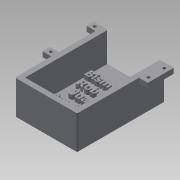
# Autodesk Inventor part: Cover Batera 2i
Saved by Autodesk Inventor 2015 SP1 (Build 190203100, 203)
## iProperties
Created: 2015-03-25
Part Number: Cover Batera 2i
Material: Generic
Document SubType Name: Modeling
Designer: Rafi Kurnia Putra
Density: 1 g/cm^3
Appearance: Default
Author: Rafi Kurnia Putra
Autodesk Inventor part; units mm, degrees
(part 1 of 2)
ref_plane "YZ Plane" through (0, 0, 0) normal (1, 0, 0) x (0, 1, 0)
ref_plane "XZ Plane" through (0, 0, 0) normal (0, 1, 0) x (-1, 0, 0)
ref_plane "XY Plane" through (0, 0, 0) normal (0, 0, 1) x (1, 0, 0)
sketch "Sketch1" plane through (0, 0, 0) normal (0, 0, 1) x (1, 0, 0)
  line L0 (-21.25, -30) -> (21.25, -30)
  line L1 (21.25, -30) -> (21.25, 30)
  line L2 (21.25, 30) -> (-21.25, 30)
  line L3 (-21.25, 30) -> (-21.25, -30)
  line L4 (-21.25, -30) -> (21.25, 30) construction
  line L5 (21.25, -30) -> (-21.25, 30) construction
  point P0 (0, 0)
  dimension "d0" = 42.5
  dimension "d1" = 60
  constraints: 12 end point, 2 midpoint, 2 parallel, 1 horizontal, 1 perpendicular
  measures "d0" distance of L2.end L1.end
  measures "d1" distance of L1.end L0.end
extrude "Extrusion1" add sketch "Sketch1" along normal blind 3.5
sketch "Sketch4" plane through (0, 0, 3.5) normal (0, 0, 1) x (1, 0, 0)
  line L0 (-21.25, -30) -> (21.25, -30) projected
  line L1 (-21.25, 30) -> (-17.75, 30)
  line L2 (-17.75, 30) -> (-17.75, -26.5)
  line L3 (-19, -30) -> (-21.25, -30)
  line L4 (-21.25, -30) -> (-21.25, 30)
  line L5 (21.25, 30) -> (17.75, 30)
  line L6 (17.75, 30) -> (17.75, -26.5)
  line L7 (19, -30) -> (21.25, -30)
  line L8 (21.25, -30) -> (21.25, 30)
  line L9 (19, -30) -> (-19, -30)
  line L10 (-17.75, -26.5) -> (17.75, -26.5)
  point P0 (0, 0)
  dimension "d23" = 3.5
  constraints: 20 end point, 5 parallel, 4 horizontal, 3 vertical, 2 perpendicular, 2 point on line
  measures "d23" distance between parallel lines of L8 L6
extrude "Extrusion3" add sketch "Sketch4" along normal blind 20
sketch "Sketch5" plane through (0, 0, 23.5) normal (0, 0, 1) x (1, 0, 0)
  line L0 (-21.25, 30) -> (-27.25, 30)
  line L1 (-27.25, 30) -> (-27.25, -30)
  line L2 (-27.25, -30) -> (-21.25, -30)
  line L3 (-21.25, -30) -> (-21.25, 30)
  line L4 (21.25, 30) -> (27.25, 30)
  line L5 (27.25, 30) -> (27.25, -30)
  line L6 (27.25, -30) -> (21.25, -30)
  line L7 (21.25, -30) -> (21.25, 30)
  point P0 (0, 0)
  dimension "d21" = 6
  dimension "d22" = 6
  constraints: 16 end point, 4 parallel, 2 horizontal, 2 perpendicular, 1 point on line
  measures "d21" distance of L4.start L4.end
  measures "d22" distance of L0.start L0.end
extrude "Extrusion4" add sketch "Sketch5" against normal blind 3.5
sketch "Sketch6" plane through (0, 0, 20) normal (0, 0, -1) x (-1, 0, 0)
  line L0 (-27.25, 30) -> (-27.25, -30) projected
  line L1 (-21.25, -30) -> (-21.25, 30) projected
  line L2 (-27.25, 25) -> (-21.25, 25)
  line L3 (-21.25, 25) -> (-21.25, 0)
  line L4 (-21.25, 0) -> (-27.25, 0)
  line L5 (-27.25, 0) -> (-27.25, 25)
  point P0 (0, 0)
  constraints: 8 end point, 2 parallel, 1 horizontal, 1 midpoint, 1 perpendicular, 1 point on line
extrude "Extrusion5" cut sketch "Sketch6" against normal up to next
sketch "Sketch7" plane through (0, 0, 20) normal (0, 0, -1) x (-1, 0, 0)
  line L0 (21.25, 12.215) -> (41.1215, 12.215) projected
  line L1 (27.25, -30) -> (27.25, 30) projected
  line L2 (27.25, 12.215) -> (21.25, 12.215)
  line L3 (21.25, 12.215) -> (21.25, -30)
  line L4 (21.25, -30) -> (27.25, -30)
  line L5 (27.25, -30) -> (27.25, 12.215)
  point P0 (0, 0)
  constraints: 8 end point, 2 parallel, 2 point on line, 1 horizontal, 1 perpendicular
extrude "Extrusion6" cut sketch "Sketch7" against normal up to next
sketch "Sketch8" plane through (0, 0, 20) normal (0, 0, -1) x (-1, 0, 0)
  line L0 (-29.9641, -5.0076) -> (-82.628, -5.0076) projected
  line L1 (-27.25, 0) -> (-27.25, -30) projected
  line L2 (-27.25, -5.0076) -> (-21.25, -5.0076)
  line L3 (-21.25, -5.0076) -> (-21.25, -30)
  line L4 (-21.25, -30) -> (-27.25, -30)
  line L5 (-27.25, -30) -> (-27.25, -5.0076)
  point P0 (0, 0)
  constraints: 8 end point, 2 parallel, 1 horizontal, 1 perpendicular, 1 point on line
extrude "Extrusion7" cut sketch "Sketch8" against normal up to next
sketch "Sketch11" plane through (0, 0, 20) normal (0, 0, -1) x (-1, 0, 0)
  line L0 (-27.25, 25) -> (-21.25, 25) projected
  line L1 (-21.25, 30) -> (-21.25, 25) projected
  line L2 (-21.25, 30) -> (-27.25, 30) projected
  line L3 (-27.25, 30) -> (-27.25, 25) projected
  line L4 (-27.25, -5.0076) -> (-21.25, -5.0076) projected
  line L5 (-21.25, 0) -> (-21.25, -5.0076) projected
  line L6 (-21.25, 0) -> (-27.25, 0) projected
  line L7 (-27.25, 0) -> (-27.25, -5.0076) projected
  line L8 (21.25, 12.215) -> (27.25, 12.215) projected
  line L9 (27.25, 12.215) -> (27.25, 30) projected
  line L10 (27.25, 30) -> (21.25, 30) projected
  line L11 (21.25, 12.215) -> (21.25, 30) projected
  circle A0 centre (-24.25, 27.5) radius 1
  circle A1 centre (-24.25, -2.5038) radius 1
  circle A2 centre (24.25, 26.5) radius 1
  circle A3 centre (24.25, 15.715) radius 1
  point P0 (0, 0)
  dimension "d24" = 2
  dimension "d25" = 2
  dimension "d26" = 2
  dimension "d27" = 2
  dimension "d28" = 3.5
  constraints: 4 centre point
  measures "d24" diameter of A0
  measures "d25" diameter of A1
  measures "d26" diameter of A2
  measures "d27" diameter of A3
  measures "d28" distance from line of L8 A3.centre
extrude "Extrusion8" cut sketch "Sketch11" against normal up to next contours A0 | A1 | A2 | A3
fillet "Fillet1" radius 1 8 edges at (-21.25, 0, 0) (21.25, 0, 0) (0, -30, 0) (-21.25, -30, 11.75) (21.25, -30, 11.75) (0, 30, 0) (-21.25, 30, 10) (21.25, 30, 10)
sketch "Sketch12" plane through (0, 0, 0) normal (0, 0, -1) x (-1, 0, 0)
  line L0 (-18.2931, -19.3693) -> (18.2839, -19.3693) construction
  line L1 (18.2839, -19.3693) -> (18.2839, -25.7267) construction
  line L2 (18.2839, -25.7267) -> (-18.2931, -25.7267) construction
  line L3 (-18.2931, -25.7267) -> (-18.2931, -19.3693) construction
  line L4 (-11.5666, -25.048) -> (-13.0942, -25.048)
  line L5 (-13.0942, -25.048) -> (-14.484, -23.2125)
  line L6 (-14.484, -23.2125) -> (-14.9378, -23.2125)
  line L7 (-14.9378, -23.2125) -> (-14.9378, -25.048)
  line L8 (-14.9378, -25.048) -> (-16.1858, -25.048)
  line L9 (-16.1858, -25.048) -> (-16.1858, -20.048)
  line L10 (-16.1858, -20.048) -> (-14.176, -20.048)
  spline S0 degree 2 poles (-14.176, -20.048) (-13.7587, -20.048) (-13.1428, -20.1533) (-12.8794, -20.3154) knots 0 0 0 1 2 2 2
  spline S1 degree 2 poles (-12.8794, -20.3154) (-12.612, -20.4856) (-12.296, -21.0164) (-12.296, -21.4216) knots 0 0 0 1 2 2 2
  spline S2 degree 2 poles (-12.296, -21.4216) (-12.296, -21.9929) (-12.8146, -22.7101) (-13.2482, -22.9208) knots 0 0 0 1 2 2 2
  line L11 (-13.2482, -22.9208) -> (-11.5666, -25.048)
  spline S3 degree 2 poles (-13.5845, -21.5796) (-13.5845, -21.3892) (-13.7303, -21.1177) (-13.8965, -21.0447) knots 0 0 0 1 2 2 2
  spline S4 degree 2 poles (-13.8965, -21.0447) (-14.014, -20.9961) (-14.3016, -20.9678) (-14.5164, -20.9678) knots 0 0 0 1 2 2 2
  line L12 (-14.5164, -20.9678) -> (-14.9378, -20.9678)
  line L13 (-14.9378, -20.9678) -> (-14.9378, -22.313)
  line L14 (-14.9378, -22.313) -> (-14.5772, -22.313)
  spline S5 degree 2 poles (-14.5772, -22.313) (-14.3178, -22.313) (-13.9491, -22.2482) (-13.8235, -22.1469) knots 0 0 0 1 2 2 2
  spline S6 degree 2 poles (-13.8235, -22.1469) (-13.702, -22.0496) (-13.5845, -21.7903) (-13.5845, -21.5796) knots 0 0 0 1 2 2 2
  spline S7 degree 2 poles (-6.6436, -22.548) (-6.6436, -23.7636) (-7.9402, -25.1533) (-9.0666, -25.1533) knots 0 0 0 1 2 2 2
  spline S8 degree 2 poles (-9.0666, -25.1533) (-10.1971, -25.1533) (-11.4856, -23.7473) (-11.4856, -22.548) knots 0 0 0 1 2 2 2
  spline S9 degree 2 poles (-11.4856, -22.548) (-11.4856, -21.3446) (-10.1971, -19.9426) (-9.0666, -19.9426) knots 0 0 0 1 2 2 2
  spline S10 degree 2 poles (-9.0666, -19.9426) (-7.9402, -19.9426) (-6.6436, -21.3365) (-6.6436, -22.548) knots 0 0 0 1 2 2 2
  spline S11 degree 2 poles (-7.9402, -22.548) (-7.9402, -22.0982) (-8.1225, -21.4702) (-8.2806, -21.2717) knots 0 0 0 1 2 2 2
  spline S12 degree 2 poles (-8.2806, -21.2717) (-8.4386, -21.065) (-8.8438, -20.8867) (-9.0626, -20.8867) knots 0 0 0 1 2 2 2
  spline S13 degree 2 poles (-9.0626, -20.8867) (-9.2935, -20.8867) (-9.6704, -21.0529) (-9.8446, -21.2636) knots 0 0 0 1 2 2 2
  spline S14 degree 2 poles (-9.8446, -21.2636) (-9.9986, -21.458) (-10.189, -22.1023) (-10.189, -22.548) knots 0 0 0 1 2 2 2
  spline S15 degree 2 poles (-10.189, -22.548) (-10.189, -23.0099) (-10.0067, -23.6177) (-9.8486, -23.8243) knots 0 0 0 1 2 2 2
  spline S16 degree 2 poles (-9.8486, -23.8243) (-9.6906, -24.031) (-9.2814, -24.2093) (-9.0626, -24.2093) knots 0 0 0 1 2 2 2
  spline S17 degree 2 poles (-9.0626, -24.2093) (-8.8397, -24.2093) (-8.4264, -24.0188) (-8.2765, -23.8162) knots 0 0 0 1 2 2 2
  spline S18 degree 2 poles (-8.2765, -23.8162) (-8.1144, -23.5974) (-7.9402, -23.018) (-7.9402, -22.548) knots 0 0 0 1 2 2 2
  spline S19 degree 2 poles (-1.9029, -23.5164) (-1.9029, -23.8892) (-2.1866, -24.4524) (-2.4216, -24.6388) knots 0 0 0 1 2 2 2
  spline S20 degree 2 poles (-2.4216, -24.6388) (-2.7052, -24.8616) (-3.3778, -25.048) (-3.9005, -25.048) knots 0 0 0 1 2 2 2
  line L15 (-3.9005, -25.048) -> (-5.8981, -25.048)
  line L16 (-5.8981, -25.048) -> (-5.8981, -20.048)
  line L17 (-5.8981, -20.048) -> (-4.1355, -20.048)
  spline S21 degree 2 poles (-4.1355, -20.048) (-3.5845, -20.048) (-3.0172, -20.1331) (-2.77, -20.2668) knots 0 0 0 1 2 2 2
  spline S22 degree 2 poles (-2.77, -20.2668) (-2.4986, -20.4086) (-2.2352, -20.8948) (-2.2352, -21.2109) knots 0 0 0 1 2 2 2
  spline S23 degree 2 poles (-2.2352, -21.2109) (-2.2352, -21.5755) (-2.5999, -22.1469) (-2.924, -22.2806) knots 0 0 0 1 2 2 2
  line L18 (-2.924, -22.2806) -> (-2.924, -22.3049)
  spline S24 degree 2 poles (-2.924, -22.3049) (-2.458, -22.4021) (-1.9029, -23.0059) (-1.9029, -23.5164) knots 0 0 0 1 2 2 2
  spline S25 degree 2 poles (-3.1995, -23.4961) (-3.1995, -23.2611) (-3.3859, -22.9977) (-3.5723, -22.9289) knots 0 0 0 1 2 2 2
  spline S26 degree 2 poles (-3.5723, -22.9289) (-3.6858, -22.8843) (-4.0869, -22.8762) (-4.4191, -22.8762) knots 0 0 0 1 2 2 2
  line L19 (-4.4191, -22.8762) -> (-4.6501, -22.8762)
  line L20 (-4.6501, -22.8762) -> (-4.6501, -24.1363)
  line L21 (-4.6501, -24.1363) -> (-4.5812, -24.1363)
  spline S27 degree 2 poles (-4.5812, -24.1363) (-4.095, -24.1363) (-3.7222, -24.1242) (-3.5277, -24.0391) knots 0 0 0 1 2 2 2
  spline S28 degree 2 poles (-3.5277, -24.0391) (-3.3576, -23.9621) (-3.1995, -23.6785) (-3.1995, -23.4961) knots 0 0 0 1 2 2 2
  spline S29 degree 2 poles (-3.5115, -21.458) (-3.5115, -21.3365) (-3.6371, -21.0812) (-3.7668, -21.0245) knots 0 0 0 1 2 2 2
  spline S30 degree 2 poles (-3.7668, -21.0245) (-3.8883, -20.9678) (-4.2287, -20.9597) (-4.565, -20.9597) knots 0 0 0 1 2 2 2
  line L22 (-4.565, -20.9597) -> (-4.6501, -20.9597)
  line L23 (-4.6501, -20.9597) -> (-4.6501, -22.0212)
  line L24 (-4.6501, -22.0212) -> (-4.4921, -22.0212)
  spline S31 degree 2 poles (-4.4921, -22.0212) (-4.172, -22.0212) (-3.9127, -22.0091) (-3.7749, -21.9443) knots 0 0 0 1 2 2 2
  spline S32 degree 2 poles (-3.7749, -21.9443) (-3.625, -21.8713) (-3.5115, -21.6242) (-3.5115, -21.458) knots 0 0 0 1 2 2 2
  spline S33 degree 2 poles (0.8402, -25.1533) (-0.1687, -25.1533) (-1.2546, -24.1809) (-1.2546, -23.2409) knots 0 0 0 1 2 2 2
  line L25 (-1.2546, -23.2409) -> (-1.2546, -20.048)
  line L26 (-1.2546, -20.048) -> (0.0014, -20.048)
  line L27 (0.0014, -20.048) -> (0.0014, -23.1679)
  spline S34 degree 2 poles (0.0014, -23.1679) (0.0014, -23.6906) (0.3945, -24.2012) (0.8402, -24.2012) knots 0 0 0 1 2 2 2
  spline S35 degree 2 poles (0.8402, -24.2012) (1.2737, -24.2012) (1.6789, -23.7109) (1.6789, -23.1679) knots 0 0 0 1 2 2 2
  line L28 (1.6789, -23.1679) -> (1.6789, -20.048)
  line L29 (1.6789, -20.048) -> (2.935, -20.048)
  line L30 (2.935, -20.048) -> (2.935, -23.2368)
  spline S36 degree 2 poles (2.935, -23.2368) (2.935, -24.1606) (1.8775, -25.1533) (0.8402, -25.1533) knots 0 0 0 1 2 2 2
  spline S37 degree 2 poles (5.4431, -25.1371) (4.8677, -25.1371) (4.0006, -24.9143) (3.6279, -24.7522) knots 0 0 0 1 2 2 2
  line L31 (3.6279, -24.7522) -> (3.6279, -23.561)
  line L32 (3.6279, -23.561) -> (3.7413, -23.561)
  spline S38 degree 2 poles (3.7413, -23.561) (4.1181, -23.8811) (5.0217, -24.2255) (5.4471, -24.2255) knots 0 0 0 1 2 2 2
  spline S39 degree 2 poles (5.4471, -24.2255) (5.5565, -24.2255) (5.9091, -24.1768) (6.0144, -24.1282) knots 0 0 0 1 2 2 2
  spline S40 degree 2 poles (6.0144, -24.1282) (6.1441, -24.0715) (6.3264, -23.8648) (6.3264, -23.6987) knots 0 0 0 1 2 2 2
  spline S41 degree 2 poles (6.3264, -23.6987) (6.3264, -23.5083) (6.0306, -23.2733) (5.828, -23.2206) knots 0 0 0 1 2 2 2
  spline S42 degree 2 poles (5.828, -23.2206) (5.5728, -23.1517) (4.9933, -23.0342) (4.7381, -22.9451) knots 0 0 0 1 2 2 2
  spline S43 degree 2 poles (4.7381, -22.9451) (4.1587, -22.7425) (3.6562, -22.0496) (3.6562, -21.531) knots 0 0 0 1 2 2 2
  spline S44 degree 2 poles (3.6562, -21.531) (3.6562, -20.83) (4.8434, -19.9589) (5.7348, -19.9589) knots 0 0 0 1 2 2 2
  spline S45 degree 2 poles (5.7348, -19.9589) (6.1805, -19.9589) (7.0638, -20.1412) (7.4123, -20.2952) knots 0 0 0 1 2 2 2
  line L33 (7.4123, -20.2952) -> (7.4123, -21.4378)
  line L34 (7.4123, -21.4378) -> (7.3029, -21.4378)
  spline S46 degree 2 poles (7.3029, -21.4378) (7.0233, -21.1987) (6.2211, -20.8705) (5.7997, -20.8705) knots 0 0 0 1 2 2 2
  spline S47 degree 2 poles (5.7997, -20.8705) (5.6335, -20.8705) (5.3742, -20.9191) (5.2283, -20.984) knots 0 0 0 1 2 2 2
  spline S48 degree 2 poles (5.2283, -20.984) (5.1108, -21.0366) (4.9407, -21.2473) (4.9407, -21.377) knots 0 0 0 1 2 2 2
  spline S49 degree 2 poles (4.9407, -21.377) (4.9407, -21.5715) (5.2121, -21.7943) (5.6011, -21.8835) knots 0 0 0 1 2 2 2
  spline S50 degree 2 poles (5.6011, -21.8835) (5.8523, -21.9402) (6.3183, -22.0496) (6.5857, -22.1428) knots 0 0 0 1 2 2 2
  spline S51 degree 2 poles (6.5857, -22.1428) (7.1044, -22.3332) (7.6108, -22.9653) (7.6108, -23.484) knots 0 0 0 1 2 2 2
  spline S52 degree 2 poles (7.6108, -23.484) (7.6108, -24.2295) (6.4399, -25.1371) (5.4431, -25.1371) knots 0 0 0 1 2 2 2
  line L35 (9.2154, -25.048) -> (9.2154, -21.0002)
  line L36 (9.2154, -21.0002) -> (7.7365, -21.0002)
  line L37 (7.7365, -21.0002) -> (7.7365, -20.048)
  line L38 (7.7365, -20.048) -> (11.9504, -20.048)
  line L39 (11.9504, -20.048) -> (11.9504, -21.0002)
  line L40 (11.9504, -21.0002) -> (10.4715, -21.0002)
  line L41 (10.4715, -21.0002) -> (10.4715, -25.048)
  line L42 (10.4715, -25.048) -> (9.2154, -25.048)
  line L43 (11.9261, -25.048) -> (13.6157, -20.048)
  line L44 (13.6157, -20.048) -> (14.9852, -20.048)
  line L45 (14.9852, -20.048) -> (16.6749, -25.048)
  line L46 (16.6749, -25.048) -> (15.3823, -25.048)
  line L47 (15.3823, -25.048) -> (15.0703, -24.0269)
  line L48 (15.0703, -24.0269) -> (13.4982, -24.0269)
  line L49 (13.4982, -24.0269) -> (13.1822, -25.048)
  line L50 (13.1822, -25.048) -> (11.9261, -25.048)
  line L51 (14.7948, -23.1193) -> (14.2843, -21.4661)
  line L52 (14.2843, -21.4661) -> (13.7697, -23.1193)
  line L53 (13.7697, -23.1193) -> (14.7948, -23.1193)
  point P0 (0, 0)
  constraints: 2 other
extrude "Extrusion9" cut sketch "Sketch12" against normal up to next
sketch "Sketch13" plane through (0, 0, 0) normal (0, 0, -1) x (-1, 0, 0)
  spline S0 degree 2 poles (-13.8965, -21.0447) (-14.014, -20.9961) (-14.3016, -20.9678) (-14.5164, -20.9678) knots 0 0 0 0.5 1 1 1 projected
  line L0 (-14.5164, -20.9678) -> (-14.9378, -20.9678) projected
  line L1 (-14.9378, -20.9678) -> (-14.9378, -22.313) projected
  line L2 (-14.9378, -22.313) -> (-14.5772, -22.313) projected
  spline S1 degree 2 poles (-14.5772, -22.313) (-14.3178, -22.313) (-13.9491, -22.2482) (-13.8235, -22.1469) knots 0 0 0 0.5 1 1 1 projected
  spline S2 degree 2 poles (-13.8235, -22.1469) (-13.702, -22.0496) (-13.5845, -21.7903) (-13.5845, -21.5796) knots 0 0 0 0.5 1 1 1 projected
  spline S3 degree 2 poles (-13.5845, -21.5796) (-13.5845, -21.3892) (-13.7303, -21.1177) (-13.8965, -21.0447) knots 0 0 0 0.5 1 1 1 projected
  spline S4 degree 2 poles (-8.2806, -21.2717) (-8.4386, -21.065) (-8.8438, -20.8867) (-9.0626, -20.8867) knots 0 0 0 0.5 1 1 1 projected
  spline S5 degree 2 poles (-9.0626, -20.8867) (-9.2935, -20.8867) (-9.6704, -21.0529) (-9.8446, -21.2636) knots 0 0 0 0.5 1 1 1 projected
  spline S6 degree 2 poles (-9.8446, -21.2636) (-9.9986, -21.458) (-10.189, -22.1023) (-10.189, -22.548) knots 0 0 0 0.5 1 1 1 projected
  spline S7 degree 2 poles (-10.189, -22.548) (-10.189, -23.0099) (-10.0067, -23.6177) (-9.8486, -23.8243) knots 0 0 0 0.5 1 1 1 projected
  spline S8 degree 2 poles (-9.8486, -23.8243) (-9.6906, -24.031) (-9.2814, -24.2093) (-9.0626, -24.2093) knots 0 0 0 0.5 1 1 1 projected
  spline S9 degree 2 poles (-9.0626, -24.2093) (-8.8397, -24.2093) (-8.4264, -24.0188) (-8.2765, -23.8162) knots 0 0 0 0.5 1 1 1 projected
  spline S10 degree 2 poles (-8.2765, -23.8162) (-8.1144, -23.5974) (-7.9402, -23.018) (-7.9402, -22.548) knots 0 0 0 0.5 1 1 1 projected
  spline S11 degree 2 poles (-7.9402, -22.548) (-7.9402, -22.0982) (-8.1225, -21.4702) (-8.2806, -21.2717) knots 0 0 0 0.5 1 1 1 projected
  spline S12 degree 2 poles (-3.7668, -21.0245) (-3.8883, -20.9678) (-4.2287, -20.9597) (-4.565, -20.9597) knots 0 0 0 0.5 1 1 1 projected
  line L3 (-4.565, -20.9597) -> (-4.6501, -20.9597) projected
  line L4 (-4.6501, -20.9597) -> (-4.6501, -22.0212) projected
  line L5 (-4.6501, -22.0212) -> (-4.4921, -22.0212) projected
  spline S13 degree 2 poles (-4.4921, -22.0212) (-4.172, -22.0212) (-3.9127, -22.0091) (-3.7749, -21.9443) knots 0 0 0 0.5 1 1 1 projected
  spline S14 degree 2 poles (-3.7749, -21.9443) (-3.625, -21.8713) (-3.5115, -21.6242) (-3.5115, -21.458) knots 0 0 0 0.5 1 1 1 projected
  spline S15 degree 2 poles (-3.5115, -21.458) (-3.5115, -21.3365) (-3.6371, -21.0812) (-3.7668, -21.0245) knots 0 0 0 0.5 1 1 1 projected
  spline S16 degree 2 poles (-3.5723, -22.9289) (-3.6858, -22.8843) (-4.0869, -22.8762) (-4.4191, -22.8762) knots 0 0 0 0.5 1 1 1 projected
  line L6 (-4.4191, -22.8762) -> (-4.6501, -22.8762) projected
  line L7 (-4.6501, -22.8762) -> (-4.6501, -24.1363) projected
  line L8 (-4.6501, -24.1363) -> (-4.5812, -24.1363) projected
  spline S17 degree 2 poles (-4.5812, -24.1363) (-4.095, -24.1363) (-3.7222, -24.1242) (-3.5277, -24.0391) knots 0 0 0 0.5 1 1 1 projected
  spline S18 degree 2 poles (-3.5277, -24.0391) (-3.3576, -23.9621) (-3.1995, -23.6785) (-3.1995, -23.4961) knots 0 0 0 0.5 1 1 1 projected
  spline S19 degree 2 poles (-3.1995, -23.4961) (-3.1995, -23.2611) (-3.3859, -22.9977) (-3.5723, -22.9289) knots 0 0 0 0.5 1 1 1 projected
  line L9 (14.2843, -21.4661) -> (13.7697, -23.1193) projected
  line L10 (13.7697, -23.1193) -> (14.7948, -23.1193) projected
  line L11 (14.7948, -23.1193) -> (14.2843, -21.4661) projected
  point P0 (0, 0)
  constraints: 20 other
extrude "Extrusion10" cut sketch "Sketch13" against normal up to next
fillet "Fillet2" radius 1 3 edges at (-17.75, 30, 13.5) (0, 30, 3.5) (17.75, 30, 13.5)
sketch "Sketch15" plane through (0, 0, 23.5) normal (0, 0, 1) x (1, 0, 0)
  circle A0 centre (-24.25, 15.715) radius 1 projected
  circle A1 centre (24.25, -2.5038) radius 1 projected
  circle A2 centre (24.25, 27.5) radius 1 projected
  circle A3 centre (-24.25, 26.5) radius 1 projected
  arc A4 (18.75, 30) -> (17.75, 29) centre (18.75, 29) ccw projected
  line L0 (17.75, 29) -> (17.75, -26.5) projected
  line L1 (17.75, -26.5) -> (-17.75, -26.5) projected
  line L2 (-17.75, -26.5) -> (-17.75, 29) projected
  arc A5 (-17.75, 29) -> (-18.75, 30) centre (-18.75, 29) ccw projected
  line L3 (-18.75, 30) -> (-27.25, 30) projected
  line L4 (-27.25, 30) -> (-27.25, 12.215) projected
  line L5 (-27.25, 12.215) -> (-21.25, 12.215) projected
  line L6 (-21.25, 12.215) -> (-21.25, -29) projected
  arc A6 (-21.25, -29) -> (-20.25, -30) centre (-20.25, -29) ccw projected
  line L7 (-20.25, -30) -> (20.25, -30) projected
  arc A7 (20.25, -30) -> (21.25, -29) centre (20.25, -29) ccw projected
  line L8 (21.25, -29) -> (21.25, -5.0076) projected
  line L9 (21.25, -5.0076) -> (27.25, -5.0076) projected
  line L10 (27.25, 0) -> (27.25, -5.0076) projected
  line L11 (27.25, 0) -> (21.25, 0) projected
  line L12 (21.25, 0) -> (21.25, 25) projected
  line L13 (21.25, 25) -> (27.25, 25) projected
  line L14 (27.25, 30) -> (27.25, 25) projected
  line L15 (18.75, 30) -> (27.25, 30) projected
  point P0 (0, 0)
extrude "Extrusion11" cut sketch "Sketch15" against normal blind 3.5
sketch "Sketch16" plane through (0, 0, 20) normal (0, 0, 1) x (1, 0, 0)
  line L0 (-27.25, 0) -> (-21.25, 0)
  line L1 (-21.25, -5.0076) -> (-27.25, -5.0076)
  line L2 (-27.25, 0) -> (-27.25, -5.0076)
  circle A0 centre (-24.25, -2.5038) radius 1
  line L3 (-21.25, 0) -> (-21.25, 25)
  line L4 (-17.75, 29) -> (-17.75, -26.5)
  line L5 (17.75, -26.5) -> (17.75, 29)
  line L6 (-21.25, -29) -> (-21.25, -5.0076)
  arc A1 (-21.25, -29) -> (-20.25, -30) centre (-20.25, -29) ccw
  line L7 (21.25, 12.215) -> (21.25, -29)
  line L8 (-17.75, -26.5) -> (17.75, -26.5)
  line L9 (20.25, -30) -> (-20.25, -30)
  arc A2 (-17.75, 29) -> (-18.75, 30) centre (-18.75, 29) ccw
  line L10 (-21.25, 25) -> (-27.25, 25)
  circle A3 centre (-24.25, 27.5) radius 1
  line L11 (-18.75, 30) -> (-27.25, 30)
  line L12 (-27.25, 30) -> (-27.25, 25)
  arc A4 (20.25, -30) -> (21.25, -29) centre (20.25, -29) ccw
  circle A5 centre (24.25, 26.5) radius 1
  circle A6 centre (24.25, 15.715) radius 1
  line L13 (27.25, 12.215) -> (21.25, 12.215)
  line L14 (27.25, 30) -> (27.25, 12.215)
  line L15 (18.75, 30) -> (27.25, 30)
  arc A7 (18.75, 30) -> (17.75, 29) centre (18.75, 29) ccw
  point P0 (0, 0)
  constraints: 32 end point, 8 centre point, 8 point on circle
extrude "Extrusion12" add sketch "Sketch16" along normal blind 3.5
sketch "Sketch17" plane through (17.75, -26.5, 3.5) normal (-1, 0, 0) x (0, 0, 1)
  point P0 (-3.5, 26.5)
sketch "Sketch19" plane through (0, 0, 3.5) normal (0, 0, 1) x (1, 0, 0)
  line L0 (-10.8355, 3.968) -> (10.329, 3.968) construction
  line L1 (10.329, 3.968) -> (10.329, 0.2383) construction
  line L2 (10.329, 0.2383) -> (-10.8355, 0.2383) construction
  line L3 (-10.8355, 0.2383) -> (-10.8355, 3.968) construction
  spline S0 degree 2 poles (-12.6256, 14.0607) (-12.6256, 13.6879) (-12.9093, 13.1247) (-13.1443, 12.9383) knots 0 0 0 1 2 2 2
  spline S1 degree 2 poles (-13.1443, 12.9383) (-13.4279, 12.7155) (-14.1005, 12.5291) (-14.6232, 12.5291) knots 0 0 0 1 2 2 2
  line L4 (-14.6232, 12.5291) -> (-16.6208, 12.5291)
  line L5 (-16.6208, 12.5291) -> (-16.6208, 17.5291)
  line L6 (-16.6208, 17.5291) -> (-14.8582, 17.5291)
  spline S2 degree 2 poles (-14.8582, 17.5291) (-14.3071, 17.5291) (-13.7399, 17.444) (-13.4927, 17.3103) knots 0 0 0 1 2 2 2
  spline S3 degree 2 poles (-13.4927, 17.3103) (-13.2212, 17.1685) (-12.9579, 16.6822) (-12.9579, 16.3662) knots 0 0 0 1 2 2 2
  spline S4 degree 2 poles (-12.9579, 16.3662) (-12.9579, 16.0015) (-13.3225, 15.4302) (-13.6467, 15.2965) knots 0 0 0 1 2 2 2
  line L7 (-13.6467, 15.2965) -> (-13.6467, 15.2722)
  spline S5 degree 2 poles (-13.6467, 15.2722) (-13.1807, 15.1749) (-12.6256, 14.5712) (-12.6256, 14.0607) knots 0 0 0 1 2 2 2
  spline S6 degree 2 poles (-13.9222, 14.0809) (-13.9222, 14.316) (-14.1086, 14.5793) (-14.295, 14.6482) knots 0 0 0 1 2 2 2
  spline S7 degree 2 poles (-14.295, 14.6482) (-14.4084, 14.6928) (-14.8096, 14.7009) (-15.1418, 14.7009) knots 0 0 0 1 2 2 2
  line L8 (-15.1418, 14.7009) -> (-15.3728, 14.7009)
  line L9 (-15.3728, 14.7009) -> (-15.3728, 13.4407)
  line L10 (-15.3728, 13.4407) -> (-15.3039, 13.4407)
  spline S8 degree 2 poles (-15.3039, 13.4407) (-14.8177, 13.4407) (-14.4449, 13.4529) (-14.2504, 13.538) knots 0 0 0 1 2 2 2
  spline S9 degree 2 poles (-14.2504, 13.538) (-14.0802, 13.615) (-13.9222, 13.8986) (-13.9222, 14.0809) knots 0 0 0 1 2 2 2
  spline S10 degree 2 poles (-14.2342, 16.119) (-14.2342, 16.2406) (-14.3598, 16.4959) (-14.4895, 16.5526) knots 0 0 0 1 2 2 2
  spline S11 degree 2 poles (-14.4895, 16.5526) (-14.611, 16.6093) (-14.9514, 16.6174) (-15.2877, 16.6174) knots 0 0 0 1 2 2 2
  line L11 (-15.2877, 16.6174) -> (-15.3728, 16.6174)
  line L12 (-15.3728, 16.6174) -> (-15.3728, 15.5558)
  line L13 (-15.3728, 15.5558) -> (-15.2148, 15.5558)
  spline S12 degree 2 poles (-15.2148, 15.5558) (-14.8947, 15.5558) (-14.6353, 15.568) (-14.4976, 15.6328) knots 0 0 0 1 2 2 2
  spline S13 degree 2 poles (-14.4976, 15.6328) (-14.3477, 15.7057) (-14.2342, 15.9529) (-14.2342, 16.119) knots 0 0 0 1 2 2 2
  line L14 (-10.7982, 12.5291) -> (-11.9733, 12.5291)
  line L15 (-11.9733, 12.5291) -> (-11.9733, 16.3014)
  line L16 (-11.9733, 16.3014) -> (-10.7982, 16.3014)
  line L17 (-10.7982, 16.3014) -> (-10.7982, 12.5291)
  line L18 (-10.7618, 16.8403) -> (-12.0057, 16.8403)
  line L19 (-12.0057, 16.8403) -> (-12.0057, 17.756)
  line L20 (-12.0057, 17.756) -> (-10.7618, 17.756)
  line L21 (-10.7618, 17.756) -> (-10.7618, 16.8403)
  spline S14 degree 2 poles (-8.752, 12.4278) (-9.1653, 12.4278) (-9.9068, 12.6101) (-10.1499, 12.7317) knots 0 0 0 1 2 2 2
  line L22 (-10.1499, 12.7317) -> (-10.1499, 13.7244)
  line L23 (-10.1499, 13.7244) -> (-10.0527, 13.7244)
  spline S15 degree 2 poles (-10.0527, 13.7244) (-9.9676, 13.6595) (-9.7529, 13.5056) (-9.5624, 13.4205) knots 0 0 0 1 2 2 2
  spline S16 degree 2 poles (-9.5624, 13.4205) (-9.3963, 13.3435) (-8.9871, 13.2341) (-8.7439, 13.2341) knots 0 0 0 1 2 2 2
  spline S17 degree 2 poles (-8.7439, 13.2341) (-8.4968, 13.2341) (-8.1159, 13.3881) (-8.1159, 13.5542) knots 0 0 0 1 2 2 2
  spline S18 degree 2 poles (-8.1159, 13.5542) (-8.1159, 13.6839) (-8.2901, 13.8216) (-8.5413, 13.8784) knots 0 0 0 1 2 2 2
  spline S19 degree 2 poles (-8.5413, 13.8784) (-8.6751, 13.9148) (-9.0843, 13.9918) (-9.2423, 14.0404) knots 0 0 0 1 2 2 2
  spline S20 degree 2 poles (-9.2423, 14.0404) (-9.688, 14.1782) (-10.1337, 14.7171) (-10.1337, 15.1587) knots 0 0 0 1 2 2 2
  spline S21 degree 2 poles (-10.1337, 15.1587) (-10.1337, 15.41) (-9.9028, 15.8557) (-9.6759, 16.0299) knots 0 0 0 1 2 2 2
  spline S22 degree 2 poles (-9.6759, 16.0299) (-9.453, 16.2001) (-8.7926, 16.4027) (-8.3752, 16.4027) knots 0 0 0 1 2 2 2
  spline S23 degree 2 poles (-8.3752, 16.4027) (-7.9781, 16.4027) (-7.3136, 16.2446) (-7.0867, 16.1352) knots 0 0 0 1 2 2 2
  line L24 (-7.0867, 16.1352) -> (-7.0867, 15.179)
  line L25 (-7.0867, 15.179) -> (-7.1799, 15.179)
  spline S24 degree 2 poles (-7.1799, 15.179) (-7.2407, 15.2276) (-7.5041, 15.3856) (-7.6256, 15.4424) knots 0 0 0 1 2 2 2
  spline S25 degree 2 poles (-7.6256, 15.4424) (-7.7755, 15.5072) (-8.1402, 15.5963) (-8.3306, 15.5963) knots 0 0 0 1 2 2 2
  spline S26 degree 2 poles (-8.3306, 15.5963) (-8.5859, 15.5963) (-8.9384, 15.4221) (-8.9384, 15.2803) knots 0 0 0 1 2 2 2
  spline S27 degree 2 poles (-8.9384, 15.2803) (-8.9384, 15.1506) (-8.7642, 15.0048) (-8.4725, 14.9318) knots 0 0 0 1 2 2 2
  spline S28 degree 2 poles (-8.4725, 14.9318) (-8.3225, 14.8954) (-7.9295, 14.8265) (-7.7472, 14.7657) knots 0 0 0 1 2 2 2
  spline S29 degree 2 poles (-7.7472, 14.7657) (-7.342, 14.636) (-6.9206, 14.1296) (-6.9206, 13.7082) knots 0 0 0 1 2 2 2
  spline S30 degree 2 poles (-6.9206, 13.7082) (-6.9206, 13.4448) (-7.1678, 12.9626) (-7.3987, 12.8006) knots 0 0 0 1 2 2 2
  spline S31 degree 2 poles (-7.3987, 12.8006) (-7.6378, 12.6223) (-8.2942, 12.4278) (-8.752, 12.4278) knots 0 0 0 1 2 2 2
  line L26 (-1.8598, 12.5291) -> (-1.8598, 14.4132)
  spline S32 degree 2 poles (-1.8598, 14.4132) (-1.8598, 14.6928) (-1.8801, 15.0737) (-1.9287, 15.1952) knots 0 0 0 1 2 2 2
  spline S33 degree 2 poles (-1.9287, 15.1952) (-1.9814, 15.3168) (-2.1921, 15.4262) (-2.3825, 15.4262) knots 0 0 0 1 2 2 2
  spline S34 degree 2 poles (-2.3825, 15.4262) (-2.5162, 15.4262) (-2.7755, 15.3087) (-2.9295, 15.1993) knots 0 0 0 1 2 2 2
  line L27 (-2.9295, 15.1993) -> (-2.9295, 12.5291)
  line L28 (-2.9295, 12.5291) -> (-4.1127, 12.5291)
  line L29 (-4.1127, 12.5291) -> (-4.1127, 14.4132)
  spline S35 degree 2 poles (-4.1127, 14.4132) (-4.1127, 14.6887) (-4.137, 15.0737) (-4.1856, 15.1952) knots 0 0 0 1 2 2 2
  spline S36 degree 2 poles (-4.1856, 15.1952) (-4.2383, 15.3168) (-4.449, 15.4262) (-4.6394, 15.4262) knots 0 0 0 1 2 2 2
  spline S37 degree 2 poles (-4.6394, 15.4262) (-4.7812, 15.4262) (-5.0608, 15.2925) (-5.1905, 15.1993) knots 0 0 0 1 2 2 2
  line L30 (-5.1905, 15.1993) -> (-5.1905, 12.5291)
  line L31 (-5.1905, 12.5291) -> (-6.3655, 12.5291)
  line L32 (-6.3655, 12.5291) -> (-6.3655, 16.3014)
  line L33 (-6.3655, 16.3014) -> (-5.1905, 16.3014)
  line L34 (-5.1905, 16.3014) -> (-5.1905, 15.884)
  spline S38 degree 2 poles (-5.1905, 15.884) (-4.9028, 16.1271) (-4.3882, 16.4027) (-4.0681, 16.4027) knots 0 0 0 1 2 2 2
  spline S39 degree 2 poles (-4.0681, 16.4027) (-3.7237, 16.4027) (-3.1969, 16.0745) (-3.0592, 15.7463) knots 0 0 0 1 2 2 2
  spline S40 degree 2 poles (-3.0592, 15.7463) (-2.7229, 16.0623) (-2.1232, 16.4027) (-1.8153, 16.4027) knots 0 0 0 1 2 2 2
  spline S41 degree 2 poles (-1.8153, 16.4027) (-1.5519, 16.4027) (-1.1345, 16.2365) (-0.9927, 16.0664) knots 0 0 0 1 2 2 2
  spline S42 degree 2 poles (-0.9927, 16.0664) (-0.8347, 15.884) (-0.6767, 15.3856) (-0.6767, 14.9845) knots 0 0 0 1 2 2 2
  line L35 (-0.6767, 14.9845) -> (-0.6767, 12.5291)
  line L36 (-0.6767, 12.5291) -> (-1.8598, 12.5291)
  line L37 (1.3695, 12.5291) -> (0.1945, 12.5291)
  line L38 (0.1945, 12.5291) -> (0.1945, 16.3014)
  line L39 (0.1945, 16.3014) -> (1.3695, 16.3014)
  line L40 (1.3695, 16.3014) -> (1.3695, 12.5291)
  line L41 (1.406, 16.8403) -> (0.1621, 16.8403)
  line L42 (0.1621, 16.8403) -> (0.1621, 17.756)
  line L43 (0.1621, 17.756) -> (1.406, 17.756)
  line L44 (1.406, 17.756) -> (1.406, 16.8403)
  line L45 (3.4441, 12.5291) -> (2.269, 12.5291)
  line L46 (2.269, 12.5291) -> (2.269, 17.7519)
  line L47 (2.269, 17.7519) -> (3.4441, 17.7519)
  line L48 (3.4441, 17.7519) -> (3.4441, 12.5291)
  line L49 (5.5186, 12.5291) -> (4.3436, 12.5291)
  line L50 (4.3436, 12.5291) -> (4.3436, 17.7519)
  line L51 (4.3436, 17.7519) -> (5.5186, 17.7519)
  line L52 (5.5186, 17.7519) -> (5.5186, 12.5291)
  spline S43 degree 2 poles (8.4967, 12.9302) (8.3752, 12.8289) (8.1847, 12.6668) (8.0227, 12.5858) knots 0 0 0 1 2 2 2
  spline S44 degree 2 poles (8.0227, 12.5858) (7.8647, 12.5088) (7.5648, 12.4278) (7.2974, 12.4278) knots 0 0 0 1 2 2 2
  spline S45 degree 2 poles (7.2974, 12.4278) (6.795, 12.4278) (6.1345, 13.1004) (6.1345, 13.6109) knots 0 0 0 1 2 2 2
  spline S46 degree 2 poles (6.1345, 13.6109) (6.1345, 14.0283) (6.4708, 14.5469) (6.7869, 14.6968) knots 0 0 0 1 2 2 2
  spline S47 degree 2 poles (6.7869, 14.6968) (7.107, 14.8508) (7.9943, 14.9724) (8.5048, 15.0048) knots 0 0 0 1 2 2 2
  line L53 (8.5048, 15.0048) -> (8.5048, 15.025)
  spline S48 degree 2 poles (8.5048, 15.025) (8.5048, 15.337) (8.0429, 15.5761) (7.581, 15.5761) knots 0 0 0 1 2 2 2
  spline S49 degree 2 poles (7.581, 15.5761) (7.3744, 15.5761) (6.8152, 15.4262) (6.5518, 15.3087) knots 0 0 0 1 2 2 2
  line L54 (6.5518, 15.3087) -> (6.4506, 15.3087)
  line L55 (6.4506, 15.3087) -> (6.4506, 16.2203)
  spline S50 degree 2 poles (6.4506, 16.2203) (6.6248, 16.269) (7.4027, 16.4067) (7.7998, 16.4067) knots 0 0 0 1 2 2 2
  spline S51 degree 2 poles (7.7998, 16.4067) (8.7723, 16.4067) (9.6637, 15.7584) (9.6637, 15.0939) knots 0 0 0 1 2 2 2
  line L56 (9.6637, 15.0939) -> (9.6637, 12.5291)
  line L57 (9.6637, 12.5291) -> (8.4967, 12.5291)
  line L58 (8.4967, 12.5291) -> (8.4967, 12.9302)
  line L59 (8.4967, 13.5137) -> (8.4967, 14.2957)
  spline S52 degree 2 poles (8.4967, 14.2957) (8.1969, 14.2673) (7.8282, 14.2228) (7.6499, 14.1579) knots 0 0 0 1 2 2 2
  spline S53 degree 2 poles (7.6499, 14.1579) (7.4919, 14.1053) (7.3217, 13.8865) (7.3217, 13.7082) knots 0 0 0 1 2 2 2
  spline S54 degree 2 poles (7.3217, 13.7082) (7.3217, 13.4448) (7.6094, 13.2463) (7.889, 13.2463) knots 0 0 0 1 2 2 2
  spline S55 degree 2 poles (7.889, 13.2463) (8.0429, 13.2463) (8.3671, 13.3881) (8.4967, 13.5137) knots 0 0 0 1 2 2 2
  line L60 (14.064, 12.5291) -> (12.8809, 12.5291)
  line L61 (12.8809, 12.5291) -> (12.8809, 14.397)
  spline S56 degree 2 poles (12.8809, 14.397) (12.8809, 14.6279) (12.8444, 15.0818) (12.7958, 15.1871) knots 0 0 0 1 2 2 2
  spline S57 degree 2 poles (12.7958, 15.1871) (12.735, 15.3168) (12.5081, 15.4262) (12.3136, 15.4262) knots 0 0 0 1 2 2 2
  spline S58 degree 2 poles (12.3136, 15.4262) (12.1718, 15.4262) (11.876, 15.3168) (11.7099, 15.1993) knots 0 0 0 1 2 2 2
  line L62 (11.7099, 15.1993) -> (11.7099, 12.5291)
  line L63 (11.7099, 12.5291) -> (10.5348, 12.5291)
  line L64 (10.5348, 12.5291) -> (10.5348, 17.7519)
  line L65 (10.5348, 17.7519) -> (11.7099, 17.7519)
  line L66 (11.7099, 17.7519) -> (11.7099, 15.884)
  spline S59 degree 2 poles (11.7099, 15.884) (11.9976, 16.1271) (12.5446, 16.4027) (12.8768, 16.4027) knots 0 0 0 1 2 2 2
  spline S60 degree 2 poles (12.8768, 16.4027) (13.4522, 16.4027) (14.064, 15.6733) (14.064, 14.9845) knots 0 0 0 1 2 2 2
  line L67 (14.064, 14.9845) -> (14.064, 12.5291)
  line L68 (16.3614, 13.85) -> (15.1864, 11.2892)
  line L69 (15.1864, 11.2892) -> (14.4692, 11.2892)
  line L70 (14.4692, 11.2892) -> (15.1296, 13.85)
  line L71 (15.1296, 13.85) -> (16.3614, 13.85)
  line L72 (-9.3598, 4.2967) -> (-10.8874, 4.2967)
  line L73 (-10.8874, 4.2967) -> (-12.2772, 6.1322)
  line L74 (-12.2772, 6.1322) -> (-12.731, 6.1322)
  line L75 (-12.731, 6.1322) -> (-12.731, 4.2967)
  line L76 (-12.731, 4.2967) -> (-13.9789, 4.2967)
  line L77 (-13.9789, 4.2967) -> (-13.9789, 9.2967)
  line L78 (-13.9789, 9.2967) -> (-11.9692, 9.2967)
  spline S61 degree 2 poles (-11.9692, 9.2967) (-11.5519, 9.2967) (-10.936, 9.1914) (-10.6726, 9.0293) knots 0 0 0 1 2 2 2
  spline S62 degree 2 poles (-10.6726, 9.0293) (-10.4052, 8.8591) (-10.0892, 8.3283) (-10.0892, 7.9231) knots 0 0 0 1 2 2 2
  spline S63 degree 2 poles (-10.0892, 7.9231) (-10.0892, 7.3518) (-10.6078, 6.6346) (-11.0413, 6.4239) knots 0 0 0 1 2 2 2
  line L79 (-11.0413, 6.4239) -> (-9.3598, 4.2967)
  spline S64 degree 2 poles (-11.3777, 7.7651) (-11.3777, 7.9555) (-11.5235, 8.227) (-11.6896, 8.3) knots 0 0 0 1 2 2 2
  spline S65 degree 2 poles (-11.6896, 8.3) (-11.8071, 8.3486) (-12.0948, 8.3769) (-12.3096, 8.3769) knots 0 0 0 1 2 2 2
  line L80 (-12.3096, 8.3769) -> (-12.731, 8.3769)
  line L81 (-12.731, 8.3769) -> (-12.731, 7.0317)
  line L82 (-12.731, 7.0317) -> (-12.3704, 7.0317)
  spline S66 degree 2 poles (-12.3704, 7.0317) (-12.111, 7.0317) (-11.7423, 7.0965) (-11.6167, 7.1978) knots 0 0 0 1 2 2 2
  spline S67 degree 2 poles (-11.6167, 7.1978) (-11.4952, 7.2951) (-11.3777, 7.5544) (-11.3777, 7.7651) knots 0 0 0 1 2 2 2
  spline S68 degree 2 poles (-5.4376, 6.1808) (-5.4376, 5.2489) (-6.4546, 4.1792) (-7.3825, 4.1792) knots 0 0 0 1 2 2 2
  spline S69 degree 2 poles (-7.3825, 4.1792) (-8.3063, 4.1792) (-9.3315, 5.2489) (-9.3315, 6.1808) knots 0 0 0 1 2 2 2
  spline S70 degree 2 poles (-9.3315, 6.1808) (-9.3315, 7.1209) (-8.3063, 8.1865) (-7.3825, 8.1865) knots 0 0 0 1 2 2 2
  spline S71 degree 2 poles (-7.3825, 8.1865) (-6.4587, 8.1865) (-5.4376, 7.1168) (-5.4376, 6.1808) knots 0 0 0 1 2 2 2
  spline S72 degree 2 poles (-6.641, 6.1727) (-6.641, 6.509) (-6.7504, 6.9588) (-6.8477, 7.0925) knots 0 0 0 1 2 2 2
  spline S73 degree 2 poles (-6.8477, 7.0925) (-6.953, 7.2343) (-7.2164, 7.3437) (-7.3825, 7.3437) knots 0 0 0 1 2 2 2
  spline S74 degree 2 poles (-7.3825, 7.3437) (-7.5446, 7.3437) (-7.7999, 7.2465) (-7.9052, 7.1087) knots 0 0 0 1 2 2 2
  spline S75 degree 2 poles (-7.9052, 7.1087) (-8.0065, 6.979) (-8.1281, 6.5212) (-8.1281, 6.1727) knots 0 0 0 1 2 2 2
  spline S76 degree 2 poles (-8.1281, 6.1727) (-8.1281, 5.8283) (-8.0146, 5.4029) (-7.9214, 5.2732) knots 0 0 0 1 2 2 2
  spline S77 degree 2 poles (-7.9214, 5.2732) (-7.8282, 5.1436) (-7.5446, 5.022) (-7.3744, 5.022) knots 0 0 0 1 2 2 2
  spline S78 degree 2 poles (-7.3744, 5.022) (-7.2326, 5.022) (-6.9409, 5.1436) (-6.8517, 5.2651) knots 0 0 0 1 2 2 2
  spline S79 degree 2 poles (-6.8517, 5.2651) (-6.7504, 5.4069) (-6.641, 5.8162) (-6.641, 6.1727) knots 0 0 0 1 2 2 2
  spline S80 degree 2 poles (-1.1183, 6.2335) (-1.1183, 5.334) (-2.03, 4.2238) (-2.7067, 4.2238) knots 0 0 0 1 2 2 2
  spline S81 degree 2 poles (-2.7067, 4.2238) (-2.9862, 4.2238) (-3.4036, 4.3494) (-3.6386, 4.4831) knots 0 0 0 1 2 2 2
  line L83 (-3.6386, 4.4831) -> (-3.6872, 4.2967)
  line L84 (-3.6872, 4.2967) -> (-4.8136, 4.2967)
  line L85 (-4.8136, 4.2967) -> (-4.8136, 9.5196)
  line L86 (-4.8136, 9.5196) -> (-3.6386, 9.5196)
  line L87 (-3.6386, 9.5196) -> (-3.6386, 7.6719)
  spline S82 degree 2 poles (-3.6386, 7.6719) (-3.3793, 7.8948) (-2.8444, 8.1703) (-2.4919, 8.1703) knots 0 0 0 1 2 2 2
  spline S83 degree 2 poles (-2.4919, 8.1703) (-1.8315, 8.1703) (-1.1183, 7.1452) (-1.1183, 6.2335) knots 0 0 0 1 2 2 2
  spline S84 degree 2 poles (-2.3217, 6.2092) (-2.3217, 6.7724) (-2.6621, 7.2546) (-3.0187, 7.2546) knots 0 0 0 1 2 2 2
  spline S85 degree 2 poles (-3.0187, 7.2546) (-3.1767, 7.2546) (-3.4887, 7.1533) (-3.6386, 7.052) knots 0 0 0 1 2 2 2
  line L88 (-3.6386, 7.052) -> (-3.6386, 5.1638)
  spline S86 degree 2 poles (-3.6386, 5.1638) (-3.5211, 5.1152) (-3.282, 5.0828) (-3.1645, 5.0828) knots 0 0 0 1 2 2 2
  spline S87 degree 2 poles (-3.1645, 5.0828) (-2.7391, 5.0828) (-2.3217, 5.646) (-2.3217, 6.2092) knots 0 0 0 1 2 2 2
  line L89 (3.0308, 4.2967) -> (1.8557, 4.2967)
  line L90 (1.8557, 4.2967) -> (1.8557, 4.7141)
  spline S88 degree 2 poles (1.8557, 4.7141) (1.5518, 4.4588) (1.0413, 4.1914) (0.6888, 4.1914) knots 0 0 0 1 2 2 2
  spline S89 degree 2 poles (0.6888, 4.1914) (0.1296, 4.1914) (-0.4984, 4.9004) (-0.4984, 5.6136) knots 0 0 0 1 2 2 2
  line L91 (-0.4984, 5.6136) -> (-0.4984, 8.069)
  line L92 (-0.4984, 8.069) -> (0.6847, 8.069)
  line L93 (0.6847, 8.069) -> (0.6847, 6.197)
  spline S90 degree 2 poles (0.6847, 6.197) (0.6847, 5.9053) (0.7131, 5.5325) (0.7698, 5.4069) knots 0 0 0 1 2 2 2
  spline S91 degree 2 poles (0.7698, 5.4069) (0.8266, 5.2894) (1.0494, 5.1679) (1.252, 5.1679) knots 0 0 0 1 2 2 2
  spline S92 degree 2 poles (1.252, 5.1679) (1.3736, 5.1679) (1.7139, 5.2894) (1.8557, 5.3948) knots 0 0 0 1 2 2 2
  line L94 (1.8557, 5.3948) -> (1.8557, 8.069)
  line L95 (1.8557, 8.069) -> (3.0308, 8.069)
  line L96 (3.0308, 8.069) -> (3.0308, 4.2967)
  spline S93 degree 2 poles (5.077, 4.1954) (4.6637, 4.1954) (3.9222, 4.3777) (3.6791, 4.4993) knots 0 0 0 1 2 2 2
  line L97 (3.6791, 4.4993) -> (3.6791, 5.492)
  line L98 (3.6791, 5.492) -> (3.7763, 5.492)
  spline S94 degree 2 poles (3.7763, 5.492) (3.8614, 5.4272) (4.0762, 5.2732) (4.2666, 5.1881) knots 0 0 0 1 2 2 2
  spline S95 degree 2 poles (4.2666, 5.1881) (4.4327, 5.1111) (4.842, 5.0017) (5.0851, 5.0017) knots 0 0 0 1 2 2 2
  spline S96 degree 2 poles (5.0851, 5.0017) (5.3322, 5.0017) (5.7131, 5.1557) (5.7131, 5.3218) knots 0 0 0 1 2 2 2
  spline S97 degree 2 poles (5.7131, 5.3218) (5.7131, 5.4515) (5.5389, 5.5893) (5.2877, 5.646) knots 0 0 0 1 2 2 2
  spline S98 degree 2 poles (5.2877, 5.646) (5.154, 5.6824) (4.7447, 5.7594) (4.5867, 5.8081) knots 0 0 0 1 2 2 2
  spline S99 degree 2 poles (4.5867, 5.8081) (4.141, 5.9458) (3.6953, 6.4847) (3.6953, 6.9264) knots 0 0 0 1 2 2 2
  spline S100 degree 2 poles (3.6953, 6.9264) (3.6953, 7.1776) (3.9262, 7.6233) (4.1531, 7.7975) knots 0 0 0 1 2 2 2
  spline S101 degree 2 poles (4.1531, 7.7975) (4.376, 7.9677) (5.0364, 8.1703) (5.4538, 8.1703) knots 0 0 0 1 2 2 2
  spline S102 degree 2 poles (5.4538, 8.1703) (5.8509, 8.1703) (6.5154, 8.0123) (6.7423, 7.9029) knots 0 0 0 1 2 2 2
  line L99 (6.7423, 7.9029) -> (6.7423, 6.9466)
  line L100 (6.7423, 6.9466) -> (6.6491, 6.9466)
  spline S103 degree 2 poles (6.6491, 6.9466) (6.5883, 6.9953) (6.3249, 7.1533) (6.2034, 7.21) knots 0 0 0 1 2 2 2
  spline S104 degree 2 poles (6.2034, 7.21) (6.0535, 7.2748) (5.6888, 7.364) (5.4984, 7.364) knots 0 0 0 1 2 2 2
  spline S105 degree 2 poles (5.4984, 7.364) (5.2431, 7.364) (4.8906, 7.1897) (4.8906, 7.0479) knots 0 0 0 1 2 2 2
  spline S106 degree 2 poles (4.8906, 7.0479) (4.8906, 6.9183) (5.0648, 6.7724) (5.3565, 6.6995) knots 0 0 0 1 2 2 2
  spline S107 degree 2 poles (5.3565, 6.6995) (5.5065, 6.663) (5.8995, 6.5941) (6.0818, 6.5333) knots 0 0 0 1 2 2 2
  spline S108 degree 2 poles (6.0818, 6.5333) (6.487, 6.4037) (6.9084, 5.8972) (6.9084, 5.4758) knots 0 0 0 1 2 2 2
  spline S109 degree 2 poles (6.9084, 5.4758) (6.9084, 5.2124) (6.6612, 4.7303) (6.4303, 4.5682) knots 0 0 0 1 2 2 2
  spline S110 degree 2 poles (6.4303, 4.5682) (6.1912, 4.3899) (5.5348, 4.1954) (5.077, 4.1954) knots 0 0 0 1 2 2 2
  spline S111 degree 2 poles (8.91, 4.2238) (8.1929, 4.2238) (7.5364, 4.8154) (7.5364, 5.488) knots 0 0 0 1 2 2 2
  line L101 (7.5364, 5.488) -> (7.5364, 7.2505)
  line L102 (7.5364, 7.2505) -> (7.0867, 7.2505)
  line L103 (7.0867, 7.2505) -> (7.0867, 8.069)
  line L104 (7.0867, 8.069) -> (7.5364, 8.069)
  line L105 (7.5364, 8.069) -> (7.5364, 9.1468)
  line L106 (7.5364, 9.1468) -> (8.7115, 9.1468)
  line L107 (8.7115, 9.1468) -> (8.7115, 8.069)
  line L108 (8.7115, 8.069) -> (9.846, 8.069)
  line L109 (9.846, 8.069) -> (9.846, 7.2505)
  line L110 (9.846, 7.2505) -> (8.7115, 7.2505)
  line L111 (8.7115, 7.2505) -> (8.7115, 5.9094)
  spline S112 degree 2 poles (8.7115, 5.9094) (8.7115, 5.7108) (8.7196, 5.415) (8.7682, 5.2975) knots 0 0 0 1 2 2 2
  spline S113 degree 2 poles (8.7682, 5.2975) (8.8168, 5.18) (9.0559, 5.0423) (9.2828, 5.0423) knots 0 0 0 1 2 2 2
  spline S114 degree 2 poles (9.2828, 5.0423) (9.38, 5.0423) (9.6839, 5.1233) (9.7447, 5.1557) knots 0 0 0 1 2 2 2
  line L112 (9.7447, 5.1557) -> (9.846, 5.1557)
  line L113 (9.846, 5.1557) -> (9.846, 4.3291)
  spline S115 degree 2 poles (9.846, 4.3291) (9.6556, 4.2805) (9.2261, 4.2238) (8.91, 4.2238) knots 0 0 0 1 2 2 2
  spline S116 degree 2 poles (12.4027, 4.6978) (12.2812, 4.5965) (12.0907, 4.4345) (11.9287, 4.3534) knots 0 0 0 1 2 2 2
  spline S117 degree 2 poles (11.9287, 4.3534) (11.7706, 4.2765) (11.4708, 4.1954) (11.2034, 4.1954) knots 0 0 0 1 2 2 2
  spline S118 degree 2 poles (11.2034, 4.1954) (10.701, 4.1954) (10.0405, 4.868) (10.0405, 5.3786) knots 0 0 0 1 2 2 2
  spline S119 degree 2 poles (10.0405, 5.3786) (10.0405, 5.7959) (10.3768, 6.3145) (10.6929, 6.4645) knots 0 0 0 1 2 2 2
  spline S120 degree 2 poles (10.6929, 6.4645) (11.0129, 6.6184) (11.9003, 6.74) (12.4108, 6.7724) knots 0 0 0 1 2 2 2
  line L114 (12.4108, 6.7724) -> (12.4108, 6.7927)
  spline S121 degree 2 poles (12.4108, 6.7927) (12.4108, 7.1047) (11.9489, 7.3437) (11.487, 7.3437) knots 0 0 0 1 2 2 2
  spline S122 degree 2 poles (11.487, 7.3437) (11.2804, 7.3437) (10.7212, 7.1938) (10.4578, 7.0763) knots 0 0 0 1 2 2 2
  line L115 (10.4578, 7.0763) -> (10.3565, 7.0763)
  line L116 (10.3565, 7.0763) -> (10.3565, 7.988)
  spline S123 degree 2 poles (10.3565, 7.988) (10.5308, 8.0366) (11.3087, 8.1743) (11.7058, 8.1743) knots 0 0 0 1 2 2 2
  spline S124 degree 2 poles (11.7058, 8.1743) (12.6783, 8.1743) (13.5697, 7.526) (13.5697, 6.8615) knots 0 0 0 1 2 2 2
  line L117 (13.5697, 6.8615) -> (13.5697, 4.2967)
  line L118 (13.5697, 4.2967) -> (12.4027, 4.2967)
  line L119 (12.4027, 4.2967) -> (12.4027, 4.6978)
  line L120 (12.4027, 5.2813) -> (12.4027, 6.0633)
  spline S125 degree 2 poles (12.4027, 6.0633) (12.1029, 6.035) (11.7342, 5.9904) (11.5559, 5.9256) knots 0 0 0 1 2 2 2
  spline S126 degree 2 poles (11.5559, 5.9256) (11.3979, 5.8729) (11.2277, 5.6541) (11.2277, 5.4758) knots 0 0 0 1 2 2 2
  spline S127 degree 2 poles (11.2277, 5.4758) (11.2277, 5.2124) (11.5154, 5.0139) (11.795, 5.0139) knots 0 0 0 1 2 2 2
  spline S128 degree 2 poles (11.795, 5.0139) (11.9489, 5.0139) (12.2731, 5.1557) (12.4027, 5.2813) knots 0 0 0 1 2 2 2
  spline S129 degree 2 poles (-7.9741, -2.4689) (-7.9741, -2.793) (-8.1969, -3.3684) (-8.4198, -3.571) knots 0 0 0 1 2 2 2
  spline S130 degree 2 poles (-8.4198, -3.571) (-8.671, -3.7979) (-9.3558, -4.0126) (-9.8015, -4.0126) knots 0 0 0 1 2 2 2
  spline S131 degree 2 poles (-9.8015, -4.0126) (-10.1337, -4.0126) (-10.7172, -3.964) (-10.94, -3.9154) knots 0 0 0 1 2 2 2
  line L121 (-10.94, -3.9154) -> (-10.94, -2.9024)
  line L122 (-10.94, -2.9024) -> (-10.8266, -2.9024)
  spline S132 degree 2 poles (-10.8266, -2.9024) (-10.6767, -2.9632) (-10.3485, -3.0686) (-10.0892, -3.0686) knots 0 0 0 1 2 2 2
  spline S133 degree 2 poles (-10.0892, -3.0686) (-9.7569, -3.0686) (-9.3963, -2.8822) (-9.3234, -2.712) knots 0 0 0 1 2 2 2
  spline S134 degree 2 poles (-9.3234, -2.712) (-9.2464, -2.5459) (-9.2302, -2.1164) (-9.2302, -1.8489) knots 0 0 0 1 2 2 2
  line L123 (-9.2302, -1.8489) -> (-9.2302, 0.1567)
  line L124 (-9.2302, 0.1567) -> (-10.3728, 0.1567)
  line L125 (-10.3728, 0.1567) -> (-10.3728, 1.0643)
  line L126 (-10.3728, 1.0643) -> (-7.9741, 1.0643)
  line L127 (-7.9741, 1.0643) -> (-7.9741, -2.4689)
  line L128 (-3.5697, -3.9357) -> (-4.7448, -3.9357)
  line L129 (-4.7448, -3.9357) -> (-4.7448, -3.5183)
  spline S135 degree 2 poles (-4.7448, -3.5183) (-5.0486, -3.7736) (-5.5592, -4.041) (-5.9117, -4.041) knots 0 0 0 1 2 2 2
  spline S136 degree 2 poles (-5.9117, -4.041) (-6.4708, -4.041) (-7.0989, -3.3319) (-7.0989, -2.6188) knots 0 0 0 1 2 2 2
  line L130 (-7.0989, -2.6188) -> (-7.0989, -0.1634)
  line L131 (-7.0989, -0.1634) -> (-5.9157, -0.1634)
  line L132 (-5.9157, -0.1634) -> (-5.9157, -2.0353)
  spline S137 degree 2 poles (-5.9157, -2.0353) (-5.9157, -2.3271) (-5.8874, -2.6998) (-5.8306, -2.8254) knots 0 0 0 1 2 2 2
  spline S138 degree 2 poles (-5.8306, -2.8254) (-5.7739, -2.9429) (-5.5511, -3.0645) (-5.3485, -3.0645) knots 0 0 0 1 2 2 2
  spline S139 degree 2 poles (-5.3485, -3.0645) (-5.2269, -3.0645) (-4.8866, -2.9429) (-4.7448, -2.8376) knots 0 0 0 1 2 2 2
  line L133 (-4.7448, -2.8376) -> (-4.7448, -0.1634)
  line L134 (-4.7448, -0.1634) -> (-3.5697, -0.1634)
  line L135 (-3.5697, -0.1634) -> (-3.5697, -3.9357)
  spline S140 degree 2 poles (-0.5916, -3.5345) (-0.7131, -3.6358) (-0.9036, -3.7979) (-1.0657, -3.8789) knots 0 0 0 1 2 2 2
  spline S141 degree 2 poles (-1.0657, -3.8789) (-1.2237, -3.9559) (-1.5235, -4.037) (-1.7909, -4.037) knots 0 0 0 1 2 2 2
  spline S142 degree 2 poles (-1.7909, -4.037) (-2.2934, -4.037) (-2.9538, -3.3643) (-2.9538, -2.8538) knots 0 0 0 1 2 2 2
  spline S143 degree 2 poles (-2.9538, -2.8538) (-2.9538, -2.4365) (-2.6175, -1.9178) (-2.3015, -1.7679) knots 0 0 0 1 2 2 2
  spline S144 degree 2 poles (-2.3015, -1.7679) (-1.9814, -1.6139) (-1.094, -1.4924) (-0.5835, -1.46) knots 0 0 0 1 2 2 2
  line L136 (-0.5835, -1.46) -> (-0.5835, -1.4397)
  spline S145 degree 2 poles (-0.5835, -1.4397) (-0.5835, -1.1277) (-1.0454, -0.8887) (-1.5073, -0.8887) knots 0 0 0 1 2 2 2
  spline S146 degree 2 poles (-1.5073, -0.8887) (-1.714, -0.8887) (-2.2731, -1.0386) (-2.5365, -1.1561) knots 0 0 0 1 2 2 2
  line L137 (-2.5365, -1.1561) -> (-2.6378, -1.1561)
  line L138 (-2.6378, -1.1561) -> (-2.6378, -0.2444)
  spline S147 degree 2 poles (-2.6378, -0.2444) (-2.4636, -0.1958) (-1.6856, -0.058) (-1.2885, -0.058) knots 0 0 0 1 2 2 2
  spline S148 degree 2 poles (-1.2885, -0.058) (-0.3161, -0.058) (0.5753, -0.7063) (0.5753, -1.3708) knots 0 0 0 1 2 2 2
  line L139 (0.5753, -1.3708) -> (0.5753, -3.9357)
  line L140 (0.5753, -3.9357) -> (-0.5916, -3.9357)
  line L141 (-0.5916, -3.9357) -> (-0.5916, -3.5345)
  line L142 (-0.5916, -2.9511) -> (-0.5916, -2.169)
  spline S149 degree 2 poles (-0.5916, -2.169) (-0.8914, -2.1974) (-1.2601, -2.242) (-1.4384, -2.3068) knots 0 0 0 1 2 2 2
  spline S150 degree 2 poles (-1.4384, -2.3068) (-1.5965, -2.3595) (-1.7666, -2.5783) (-1.7666, -2.7566) knots 0 0 0 1 2 2 2
  spline S151 degree 2 poles (-1.7666, -2.7566) (-1.7666, -3.0199) (-1.4789, -3.2185) (-1.1994, -3.2185) knots 0 0 0 1 2 2 2
  spline S152 degree 2 poles (-1.1994, -3.2185) (-1.0454, -3.2185) (-0.7212, -3.0767) (-0.5916, -2.9511) knots 0 0 0 1 2 2 2
  line L143 (3.9789, -1.2776) -> (3.8817, -1.2776)
  spline S153 degree 2 poles (3.8817, -1.2776) (3.8128, -1.2533) (3.5575, -1.229) (3.4035, -1.229) knots 0 0 0 1 2 2 2
  spline S154 degree 2 poles (3.4035, -1.229) (3.2212, -1.229) (2.812, -1.3384) (2.6215, -1.4113) knots 0 0 0 1 2 2 2
  line L144 (2.6215, -1.4113) -> (2.6215, -3.9357)
  line L145 (2.6215, -3.9357) -> (1.4465, -3.9357)
  line L146 (1.4465, -3.9357) -> (1.4465, -0.1634)
  line L147 (1.4465, -0.1634) -> (2.6215, -0.1634)
  line L148 (2.6215, -0.1634) -> (2.6215, -0.7063)
  spline S155 degree 2 poles (2.6215, -0.7063) (2.7026, -0.6334) (2.9862, -0.4065) (3.1037, -0.3376) knots 0 0 0 1 2 2 2
  spline S156 degree 2 poles (3.1037, -0.3376) (3.2334, -0.2606) (3.5737, -0.1512) (3.7236, -0.1512) knots 0 0 0 1 2 2 2
  spline S157 degree 2 poles (3.7236, -0.1512) (3.7804, -0.1512) (3.9222, -0.1593) (3.9789, -0.1634) knots 0 0 0 1 2 2 2
  line L149 (3.9789, -0.1634) -> (3.9789, -1.2776)
  spline S158 degree 2 poles (6.5073, -3.5345) (6.3857, -3.6358) (6.1953, -3.7979) (6.0332, -3.8789) knots 0 0 0 1 2 2 2
  spline S159 degree 2 poles (6.0332, -3.8789) (5.8752, -3.9559) (5.5753, -4.037) (5.3079, -4.037) knots 0 0 0 1 2 2 2
  spline S160 degree 2 poles (5.3079, -4.037) (4.8055, -4.037) (4.145, -3.3643) (4.145, -2.8538) knots 0 0 0 1 2 2 2
  spline S161 degree 2 poles (4.145, -2.8538) (4.145, -2.4365) (4.4813, -1.9178) (4.7974, -1.7679) knots 0 0 0 1 2 2 2
  spline S162 degree 2 poles (4.7974, -1.7679) (5.1175, -1.6139) (6.0048, -1.4924) (6.5154, -1.46) knots 0 0 0 1 2 2 2
  line L150 (6.5154, -1.46) -> (6.5154, -1.4397)
  spline S163 degree 2 poles (6.5154, -1.4397) (6.5154, -1.1277) (6.0535, -0.8887) (5.5916, -0.8887) knots 0 0 0 1 2 2 2
  spline S164 degree 2 poles (5.5916, -0.8887) (5.3849, -0.8887) (4.8258, -1.0386) (4.5624, -1.1561) knots 0 0 0 1 2 2 2
  line L151 (4.5624, -1.1561) -> (4.4611, -1.1561)
  line L152 (4.4611, -1.1561) -> (4.4611, -0.2444)
  spline S165 degree 2 poles (4.4611, -0.2444) (4.6353, -0.1958) (5.4133, -0.058) (5.8104, -0.058) knots 0 0 0 1 2 2 2
  spline S166 degree 2 poles (5.8104, -0.058) (6.7828, -0.058) (7.6742, -0.7063) (7.6742, -1.3708) knots 0 0 0 1 2 2 2
  line L153 (7.6742, -1.3708) -> (7.6742, -3.9357)
  line L154 (7.6742, -3.9357) -> (6.5073, -3.9357)
  line L155 (6.5073, -3.9357) -> (6.5073, -3.5345)
  line L156 (6.5073, -2.9511) -> (6.5073, -2.169)
  spline S167 degree 2 poles (6.5073, -2.169) (6.2074, -2.1974) (5.8387, -2.242) (5.6604, -2.3068) knots 0 0 0 1 2 2 2
  spline S168 degree 2 poles (5.6604, -2.3068) (5.5024, -2.3595) (5.3322, -2.5783) (5.3322, -2.7566) knots 0 0 0 1 2 2 2